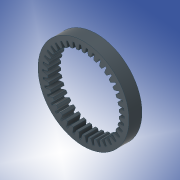
# Autodesk Inventor part: SJ011
Saved by Autodesk Inventor 2017 SP1 (Build 210196100, 196)
## iProperties
Created: 2017-07-04
Part Number: SJ011
Material: Generic
Document SubType Name: Modeling
Designer: Zach
Density: 1 g/cm^3
Appearance: CR Dark Blue
Author: Zach
Autodesk Inventor part; units mm, degrees
ref_plane "YZ Plane" through (0, 0, 0) normal (1, 0, 0) x (0, 1, 0)
ref_plane "XZ Plane" through (0, 0, 0) normal (0, 1, 0) x (-1, 0, 0)
ref_plane "XY Plane" through (0, 0, 0) normal (0, 0, 1) x (1, 0, 0)
sketch "Sketch1" plane through (0, 0, 0) normal (0, 0, 1) x (1, 0, 0)
  circle A0 centre (0, 0) radius 31.5
  circle A1 centre (0, 0) radius 35
  dimension "d0" = 63
  dimension "d27" = 70
  constraints: 2 centre point, 1 coincident
  measures "d0" diameter of A0
  measures "d27" diameter of A1
extrude "Extrusion1" add sketch "Sketch1" along normal blind 10
sketch "Sketch3" plane through (0, 0, 10) normal (0, 0, 1) x (1, 0, 0)
  circle A0 centre (0, 0) radius 27.5 construction
  line L0 (0, 0) -> (0, -31.5) construction
  circle A1 centre (0, 0) radius 31.5 construction
  arc A2 (-0.9, -27.4853) -> (-2, -31.4364) centre (12.8648, -33.4461) ccw
  arc A3 (2, -31.4364) -> (0.9, -27.4853) centre (-12.8648, -33.4461) ccw
  arc A4 (0.9, -27.4853) -> (-0.9, -27.4853) centre (0, -47.465) ccw
  arc A5 (-2, -31.4364) -> (2, -31.4364) centre (0, 0) ccw
  arc A6 (7.147, -30.6785) -> (5.4117, -26.9623) centre (-7.1843, -35.1074) ccw
  arc A7 (3.2015, -31.3369) -> (7.147, -30.6785) centre (0, 0) ccw
  arc A8 (3.6362, -27.2585) -> (3.2015, -31.3369) centre (18.1944, -30.8724) ccw
  arc A9 (5.4117, -26.9623) -> (3.6362, -27.2585) centre (7.8125, -46.8176) ccw
  arc A10 (12.099, -29.0837) -> (9.7757, -25.7038) centre (-1.3078, -35.811) ccw
  arc A11 (8.3158, -30.3825) -> (12.099, -29.0837) centre (0, 0) ccw
  arc A12 (8.0732, -26.2883) -> (8.3158, -30.3825) centre (23.0276, -27.4567) ccw
  arc A13 (9.7757, -25.7038) -> (8.0732, -26.2883) centre (15.4119, -44.8932) ccw
  arc A14 (16.721, -26.6956) -> (13.8731, -23.7442) centre (4.6043, -35.5379) ccw
  arc A15 (13.2031, -28.5994) -> (16.721, -26.6956) centre (0, 0) ccw
  arc A16 (12.29, -24.6009) -> (13.2031, -28.5994) centre (27.2328, -23.292) ccw
  arc A17 (13.8731, -23.7442) -> (12.29, -24.6009) centre (22.5908, -41.7442) ccw
  arc A18 (20.8869, -23.5793) -> (17.592, -21.1369) centre (10.3909, -34.2953) ccw
  arc A19 (17.7304, -26.0362) -> (20.8869, -23.5793) centre (0, 0) ccw
  arc A20 (16.1716, -22.2425) -> (17.7304, -26.0362) centre (30.6951, -18.4919) ccw
  arc A21 (17.592, -21.1369) -> (16.1716, -22.2425) centre (29.1536, -37.4566) ccw
  arc A22 (24.4831, -19.8199) -> (20.8311, -17.9531) centre (15.894, -32.1173) ccw
  arc A23 (21.774, -22.7628) -> (24.4831, -19.8199) centre (0, 0) ccw
  arc A24 (19.612, -19.2774) -> (21.774, -22.7628) centre (33.3201, -13.1875) ccw
  arc A25 (20.8311, -17.9531) -> (19.612, -19.2774) centre (34.9211, -32.1472) ccw
  arc A26 (27.4114, -15.5198) -> (23.502, -14.2796) centre (20.9636, -29.0632) ccw
  arc A27 (25.2236, -18.8684) -> (27.4114, -15.5198) centre (0, 0) ccw
  arc A28 (22.5175, -15.7865) -> (25.2236, -18.8684) centre (35.0363, -7.5233) ccw
  arc A29 (23.502, -14.2796) -> (22.5175, -15.7865) centre (39.7361, -25.9609) ccw
  arc A30 (29.592, -10.7963) -> (25.5318, -10.2165) centre (25.4613, -25.2163) ccw
  arc A31 (27.9853, -14.4594) -> (29.592, -10.7963) centre (0, 0) ccw
  arc A32 (24.8088, -11.8649) -> (27.9853, -14.4594) centre (35.7967, -1.6539) ccw
  arc A33 (25.5318, -10.2165) -> (24.8088, -11.8649) centre (43.4672, -19.0665) ccw
  arc A34 (30.9655, -5.7784) -> (26.8652, -5.8748) centre (29.2645, -20.6816) ccw
  arc A35 (29.9835, -9.656) -> (30.9655, -5.7784) centre (0, 0) ccw
  arc A36 (26.4233, -7.6197) -> (29.9835, -9.656) centre (35.5807, 4.2606) ccw
  arc A37 (26.8652, -5.8748) -> (26.4233, -7.6197) centre (46.0126, -11.652) ccw
  arc A38 (31.4942, -0.6028) -> (27.4657, -1.3728) centre (32.2695, -15.5828) ccw
  arc A39 (31.1639, -4.5892) -> (31.4942, -0.6028) centre (0, 0) ccw
  arc A40 (27.3171, -3.1666) -> (31.1639, -4.5892) centre (34.3942, 10.0589) ccw
  arc A41 (27.4657, -1.3728) -> (27.3171, -3.1666) centre (47.3029, -3.9196) ccw
  arc A42 (31.1639, 4.5892) -> (27.3171, 3.1666) centre (34.3942, -10.0589) ccw
  arc A43 (31.4942, 0.6028) -> (31.1639, 4.5892) centre (0, 0) ccw
  arc A44 (27.4657, 1.3728) -> (31.4942, 0.6028) centre (32.2695, 15.5828) ccw
  arc A45 (27.3171, 3.1666) -> (27.4657, 1.3728) centre (47.3029, 3.9196) ccw
  arc A46 (29.9835, 9.656) -> (26.4233, 7.6197) centre (35.5807, -4.2606) ccw
  arc A47 (30.9655, 5.7784) -> (29.9835, 9.656) centre (0, 0) ccw
  arc A48 (26.8652, 5.8748) -> (30.9655, 5.7784) centre (29.2645, 20.6816) ccw
  arc A49 (26.4233, 7.6197) -> (26.8652, 5.8748) centre (46.0126, 11.652) ccw
  arc A50 (27.9853, 14.4594) -> (24.8088, 11.8649) centre (35.7967, 1.6539) ccw
  arc A51 (29.592, 10.7963) -> (27.9853, 14.4594) centre (0, 0) ccw
  arc A52 (25.5318, 10.2165) -> (29.592, 10.7963) centre (25.4613, 25.2163) ccw
  arc A53 (24.8088, 11.8649) -> (25.5318, 10.2165) centre (43.4672, 19.0665) ccw
  arc A54 (25.2236, 18.8684) -> (22.5175, 15.7865) centre (35.0363, 7.5233) ccw
  arc A55 (27.4114, 15.5198) -> (25.2236, 18.8684) centre (0, 0) ccw
  arc A56 (23.502, 14.2796) -> (27.4114, 15.5198) centre (20.9636, 29.0632) ccw
  arc A57 (22.5175, 15.7865) -> (23.502, 14.2796) centre (39.7361, 25.9609) ccw
  arc A58 (21.774, 22.7628) -> (19.612, 19.2774) centre (33.3201, 13.1875) ccw
  arc A59 (24.4831, 19.8199) -> (21.774, 22.7628) centre (0, 0) ccw
  arc A60 (20.8311, 17.9531) -> (24.4831, 19.8199) centre (15.894, 32.1173) ccw
  arc A61 (19.612, 19.2774) -> (20.8311, 17.9531) centre (34.9211, 32.1472) ccw
  arc A62 (17.7304, 26.0362) -> (16.1716, 22.2425) centre (30.6951, 18.4919) ccw
  arc A63 (20.8869, 23.5793) -> (17.7304, 26.0362) centre (0, 0) ccw
  arc A64 (17.592, 21.1369) -> (20.8869, 23.5793) centre (10.3909, 34.2953) ccw
  arc A65 (16.1716, 22.2425) -> (17.592, 21.1369) centre (29.1536, 37.4566) ccw
  arc A66 (13.2031, 28.5994) -> (12.29, 24.6009) centre (27.2328, 23.292) ccw
  arc A67 (16.721, 26.6956) -> (13.2031, 28.5994) centre (0, 0) ccw
  arc A68 (13.8731, 23.7442) -> (16.721, 26.6956) centre (4.6043, 35.5379) ccw
  arc A69 (12.29, 24.6009) -> (13.8731, 23.7442) centre (22.5908, 41.7442) ccw
  arc A70 (8.3158, 30.3825) -> (8.0732, 26.2883) centre (23.0276, 27.4567) ccw
  arc A71 (12.099, 29.0837) -> (8.3158, 30.3825) centre (0, 0) ccw
  arc A72 (9.7757, 25.7038) -> (12.099, 29.0837) centre (-1.3078, 35.811) ccw
  arc A73 (8.0732, 26.2883) -> (9.7757, 25.7038) centre (15.4119, 44.8932) ccw
  arc A74 (3.2015, 31.3369) -> (3.6362, 27.2585) centre (18.1944, 30.8724) ccw
  arc A75 (7.147, 30.6785) -> (3.2015, 31.3369) centre (0, 0) ccw
  arc A76 (5.4117, 26.9623) -> (7.147, 30.6785) centre (-7.1843, 35.1074) ccw
  arc A77 (3.6362, 27.2585) -> (5.4117, 26.9623) centre (7.8125, 46.8176) ccw
  arc A78 (-2, 31.4364) -> (-0.9, 27.4853) centre (12.8648, 33.4461) ccw
  arc A79 (2, 31.4364) -> (-2, 31.4364) centre (0, 0) ccw
  arc A80 (0.9, 27.4853) -> (2, 31.4364) centre (-12.8648, 33.4461) ccw
  arc A81 (-0.9, 27.4853) -> (0.9, 27.4853) centre (0, 47.465) ccw
  arc A82 (-7.147, 30.6785) -> (-5.4117, 26.9623) centre (7.1843, 35.1074) ccw
  arc A83 (-3.2015, 31.3369) -> (-7.147, 30.6785) centre (0, 0) ccw
  arc A84 (-3.6362, 27.2585) -> (-3.2015, 31.3369) centre (-18.1944, 30.8724) ccw
  arc A85 (-5.4117, 26.9623) -> (-3.6362, 27.2585) centre (-7.8125, 46.8176) ccw
  arc A86 (-12.099, 29.0837) -> (-9.7757, 25.7038) centre (1.3078, 35.811) ccw
  arc A87 (-8.3158, 30.3825) -> (-12.099, 29.0837) centre (0, 0) ccw
  arc A88 (-8.0732, 26.2883) -> (-8.3158, 30.3825) centre (-23.0276, 27.4567) ccw
  arc A89 (-9.7757, 25.7038) -> (-8.0732, 26.2883) centre (-15.4119, 44.8932) ccw
  arc A90 (-16.721, 26.6956) -> (-13.8731, 23.7442) centre (-4.6043, 35.5379) ccw
  arc A91 (-13.2031, 28.5994) -> (-16.721, 26.6956) centre (0, 0) ccw
  arc A92 (-12.29, 24.6009) -> (-13.2031, 28.5994) centre (-27.2328, 23.292) ccw
  arc A93 (-13.8731, 23.7442) -> (-12.29, 24.6009) centre (-22.5908, 41.7442) ccw
  arc A94 (-20.8869, 23.5793) -> (-17.592, 21.1369) centre (-10.3909, 34.2953) ccw
  arc A95 (-17.7304, 26.0362) -> (-20.8869, 23.5793) centre (0, 0) ccw
  arc A96 (-16.1716, 22.2425) -> (-17.7304, 26.0362) centre (-30.6951, 18.4919) ccw
  arc A97 (-17.592, 21.1369) -> (-16.1716, 22.2425) centre (-29.1536, 37.4566) ccw
  arc A98 (-24.4831, 19.8199) -> (-20.8311, 17.9531) centre (-15.894, 32.1173) ccw
  arc A99 (-21.774, 22.7628) -> (-24.4831, 19.8199) centre (0, 0) ccw
  arc A100 (-19.612, 19.2774) -> (-21.774, 22.7628) centre (-33.3201, 13.1875) ccw
  arc A101 (-20.8311, 17.9531) -> (-19.612, 19.2774) centre (-34.9211, 32.1472) ccw
  arc A102 (-27.4114, 15.5198) -> (-23.502, 14.2796) centre (-20.9636, 29.0632) ccw
  arc A103 (-25.2236, 18.8684) -> (-27.4114, 15.5198) centre (0, 0) ccw
  arc A104 (-22.5175, 15.7865) -> (-25.2236, 18.8684) centre (-35.0363, 7.5233) ccw
  arc A105 (-23.502, 14.2796) -> (-22.5175, 15.7865) centre (-39.7361, 25.9609) ccw
  arc A106 (-29.592, 10.7963) -> (-25.5318, 10.2165) centre (-25.4613, 25.2163) ccw
  arc A107 (-27.9853, 14.4594) -> (-29.592, 10.7963) centre (0, 0) ccw
  arc A108 (-24.8088, 11.8649) -> (-27.9853, 14.4594) centre (-35.7967, 1.6539) ccw
  arc A109 (-25.5318, 10.2165) -> (-24.8088, 11.8649) centre (-43.4672, 19.0665) ccw
  arc A110 (-30.9655, 5.7784) -> (-26.8652, 5.8748) centre (-29.2645, 20.6816) ccw
  arc A111 (-29.9835, 9.656) -> (-30.9655, 5.7784) centre (0, 0) ccw
  arc A112 (-26.4233, 7.6197) -> (-29.9835, 9.656) centre (-35.5807, -4.2606) ccw
  arc A113 (-26.8652, 5.8748) -> (-26.4233, 7.6197) centre (-46.0126, 11.652) ccw
  arc A114 (-31.4942, 0.6028) -> (-27.4657, 1.3728) centre (-32.2695, 15.5828) ccw
  arc A115 (-31.1639, 4.5892) -> (-31.4942, 0.6028) centre (0, 0) ccw
  arc A116 (-27.3171, 3.1666) -> (-31.1639, 4.5892) centre (-34.3942, -10.0589) ccw
  arc A117 (-27.4657, 1.3728) -> (-27.3171, 3.1666) centre (-47.3029, 3.9196) ccw
  arc A118 (-31.1639, -4.5892) -> (-27.3171, -3.1666) centre (-34.3942, 10.0589) ccw
  arc A119 (-31.4942, -0.6028) -> (-31.1639, -4.5892) centre (0, 0) ccw
  arc A120 (-27.4657, -1.3728) -> (-31.4942, -0.6028) centre (-32.2695, -15.5828) ccw
  arc A121 (-27.3171, -3.1666) -> (-27.4657, -1.3728) centre (-47.3029, -3.9196) ccw
  arc A122 (-29.9835, -9.656) -> (-26.4233, -7.6197) centre (-35.5807, 4.2606) ccw
  arc A123 (-30.9655, -5.7784) -> (-29.9835, -9.656) centre (0, 0) ccw
  arc A124 (-26.8652, -5.8748) -> (-30.9655, -5.7784) centre (-29.2645, -20.6816) ccw
  arc A125 (-26.4233, -7.6197) -> (-26.8652, -5.8748) centre (-46.0126, -11.652) ccw
  arc A126 (-27.9853, -14.4594) -> (-24.8088, -11.8649) centre (-35.7967, -1.6539) ccw
  arc A127 (-29.592, -10.7963) -> (-27.9853, -14.4594) centre (0, 0) ccw
  arc A128 (-25.5318, -10.2165) -> (-29.592, -10.7963) centre (-25.4613, -25.2163) ccw
  arc A129 (-24.8088, -11.8649) -> (-25.5318, -10.2165) centre (-43.4672, -19.0665) ccw
  arc A130 (-25.2236, -18.8684) -> (-22.5175, -15.7865) centre (-35.0363, -7.5233) ccw
  arc A131 (-27.4114, -15.5198) -> (-25.2236, -18.8684) centre (0, 0) ccw
  arc A132 (-23.502, -14.2796) -> (-27.4114, -15.5198) centre (-20.9636, -29.0632) ccw
  arc A133 (-22.5175, -15.7865) -> (-23.502, -14.2796) centre (-39.7361, -25.9609) ccw
  arc A134 (-21.774, -22.7628) -> (-19.612, -19.2774) centre (-33.3201, -13.1875) ccw
  arc A135 (-24.4831, -19.8199) -> (-21.774, -22.7628) centre (0, 0) ccw
  arc A136 (-20.8311, -17.9531) -> (-24.4831, -19.8199) centre (-15.894, -32.1173) ccw
  arc A137 (-19.612, -19.2774) -> (-20.8311, -17.9531) centre (-34.9211, -32.1472) ccw
  arc A138 (-17.7304, -26.0362) -> (-16.1716, -22.2425) centre (-30.6951, -18.4919) ccw
  arc A139 (-20.8869, -23.5793) -> (-17.7304, -26.0362) centre (0, 0) ccw
  arc A140 (-17.592, -21.1369) -> (-20.8869, -23.5793) centre (-10.3909, -34.2953) ccw
  arc A141 (-16.1716, -22.2425) -> (-17.592, -21.1369) centre (-29.1536, -37.4566) ccw
  arc A142 (-13.2031, -28.5994) -> (-12.29, -24.6009) centre (-27.2328, -23.292) ccw
  arc A143 (-16.721, -26.6956) -> (-13.2031, -28.5994) centre (0, 0) ccw
  arc A144 (-13.8731, -23.7442) -> (-16.721, -26.6956) centre (-4.6043, -35.5379) ccw
  arc A145 (-12.29, -24.6009) -> (-13.8731, -23.7442) centre (-22.5908, -41.7442) ccw
  arc A146 (-8.3158, -30.3825) -> (-8.0732, -26.2883) centre (-23.0276, -27.4567) ccw
  arc A147 (-12.099, -29.0837) -> (-8.3158, -30.3825) centre (0, 0) ccw
  arc A148 (-9.7757, -25.7038) -> (-12.099, -29.0837) centre (1.3078, -35.811) ccw
  arc A149 (-8.0732, -26.2883) -> (-9.7757, -25.7038) centre (-15.4119, -44.8932) ccw
  arc A150 (-3.2015, -31.3369) -> (-3.6362, -27.2585) centre (-18.1944, -30.8724) ccw
  arc A151 (-7.147, -30.6785) -> (-3.2015, -31.3369) centre (0, 0) ccw
  arc A152 (-5.4117, -26.9623) -> (-7.147, -30.6785) centre (7.1843, -35.1074) ccw
  arc A153 (-3.6362, -27.2585) -> (-5.4117, -26.9623) centre (-7.8125, -46.8176) ccw
  point P0 (5.1847, -31.0704)
  point P1 (10.228, -29.7932)
  point P2 (14.9923, -27.7034)
  point P3 (19.3477, -24.8579)
  point P4 (23.1753, -21.3344)
  point P5 (26.3707, -17.2289)
  point P6 (28.8469, -12.6534)
  point P7 (30.5361, -7.7328)
  point P8 (31.3924, -2.6012)
  point P9 (31.3924, 2.6012)
  point P10 (30.5361, 7.7328)
  point P11 (28.8469, 12.6534)
  point P12 (26.3707, 17.2289)
  point P13 (23.1753, 21.3344)
  point P14 (19.3477, 24.8579)
  point P15 (14.9923, 27.7034)
  point P16 (10.228, 29.7932)
  point P17 (5.1847, 31.0704)
  point P18 (0, 31.5)
  point P19 (-5.1847, 31.0704)
  point P20 (-10.228, 29.7932)
  point P21 (-14.9923, 27.7034)
  point P22 (-19.3477, 24.8579)
  point P23 (-23.1753, 21.3344)
  point P24 (-26.3707, 17.2289)
  point P25 (-28.8469, 12.6534)
  point P26 (-30.5361, 7.7328)
  point P27 (-31.3924, 2.6012)
  point P28 (-31.3924, -2.6012)
  point P29 (-30.5361, -7.7328)
  point P30 (-28.8469, -12.6534)
  point P31 (-26.3707, -17.2289)
  point P32 (-23.1753, -21.3344)
  point P33 (-19.3477, -24.8579)
  point P34 (-14.9923, -27.7034)
  point P35 (-10.228, -29.7932)
  point P36 (-5.1847, -31.0704)
  dimension "d16" = 55
  dimension "d17" = 15
  dimension "d18" = 20
  dimension "d19" = 4
  dimension "d20" = 1.8
  dimension "d23" = 360
  constraints: 346 point on circle, 153 centre point, 3 symmetric about line, 2 end point, 1 coincident, 1 vertical, 496 other
  measures "d16" diameter of A0
  measures "d17" radius of A2
  measures "d18" radius of A4
  measures "d19" distance of A3.start A1.end
  measures "d20" distance of A0.end A0.start
extrude "Extrusion2" add sketch "Sketch3" against normal blind 10
body "Solid1"
